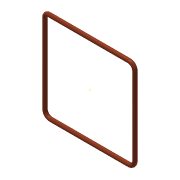
# Autodesk Inventor part: rfCoilSmaller
Saved by Autodesk Inventor 2015 (Build 190159000, 159)
## iProperties
Created: 2015-03-12
Part Number: rfCoilSmaller
Material: Generic
Document SubType Name: Modeling
Designer: jad211
Density: 1 g/cm^3
Appearance: Default
Author: jad211
Autodesk Inventor part; units mm, degrees
ref_plane "YZ Plane" through (0, 0, 0) normal (1, 0, 0) x (0, 1, 0)
ref_plane "XZ Plane" through (0, 0, 0) normal (0, 1, 0) x (-1, 0, 0)
ref_plane "XY Plane" through (0, 0, 0) normal (0, 0, 1) x (1, 0, 0)
sketch "Sketch1" plane through (0, 0, 0) normal (0, 1, 0) x (-1, 0, 0)
  line L0 (-19.5, 22.5) -> (20.5, 22.5)
  line L1 (22.5, 20.5) -> (22.5, -19.5)
  line L2 (19.5, -22.5) -> (-19.5, -22.5)
  line L3 (-22.5, -19.5) -> (-22.5, 19.5)
  line L4 (-22.5, 22.5) -> (22.5, -22.5) construction
  line L5 (22.5, 22.5) -> (-22.5, -22.5) construction
  arc A0 (22.5, 20.5) -> (20.5, 22.5) centre (20.5, 20.5) ccw
  arc A1 (19.5, -22.5) -> (22.5, -19.5) centre (19.5, -19.5) ccw
  arc A2 (-22.5, -19.5) -> (-19.5, -22.5) centre (-19.5, -19.5) ccw
  arc A3 (-19.5, 22.5) -> (-22.5, 19.5) centre (-19.5, 19.5) ccw
  point P0 (0, 0)
  dimension "d0" = 45
  dimension "d1" = 45
  dimension "d2" = 2
  dimension "d3" = 3
  constraints: 12 end point, 8 point on circle, 8 point on line, 8 tangent, 4 centre point, 2 equal radius, 2 midpoint, 2 parallel, 1 horizontal, 1 perpendicular
  measures "d0" distance of L5.start L4.end
  measures "d1" distance of L4.end L5.end
  measures "d2" radius of A0
  measures "d3" radius of A1
sketch "Sketch2" plane through (0, 0, 0) normal (0, 0, 1) x (1, 0, 0)
  point P0 (0, 0)
sketch "Sketch3" plane through (0, 0, 0) normal (0, 0, 1) x (1, 0, 0)
  circle A0 centre (22.5, 0) radius 0.9712
  point P0 (0, 0)
  dimension "d5" = 22.5
  constraints: 1 centre point
  measures "d5" distance of point (0, 0) A0.centre
sweep "Sweep1" add profiles "Sketch3" path "Sketch1"
equation "\"d1\" = d0"
equation "\"d5\" = 0.5 * d1"
body "Solid1"
